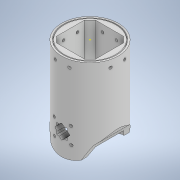
# Autodesk Inventor part: brazo_base_1
Saved by Autodesk Inventor 2021 (Build 250183000, 183)
## iProperties
Created: 2021-03-15
Part Number: brazo_base_1
Material: Genérico
Document SubType Name: Modeling
Designer: Joaquín
Density: 1 g/cm^3
Appearance: Valor por defecto
Author: Joaquín
Autodesk Inventor part; units mm, degrees
ref_plane "YZ Plane" through (0, 0, 0) normal (1, 0, 0) x (0, 1, 0)
ref_plane "XZ Plane" through (0, 0, 0) normal (0, 1, 0) x (-1, 0, 0)
ref_plane "XY Plane" through (0, 0, 0) normal (0, 0, 1) x (1, 0, 0)
sketch "Boceto4" plane through (0, 0, 0) normal (0, 1, 0) x (-1, 0, 0)
  line L0 (-22.5, 0) -> (-22.5, -16)
  line L1 (0, -22.5) -> (-16, -22.5)
  line L2 (-16, -22.5) -> (-22.5, -16)
  line L3 (0, -22.5) -> (16, -22.5)
  line L4 (22.5, 0) -> (22.5, -16)
  line L5 (22.5, -16) -> (16, -22.5)
  line L6 (22.5, 0) -> (22.5, 16)
  line L7 (0, 22.5) -> (16, 22.5)
  line L8 (16, 22.5) -> (22.5, 16)
  line L9 (0, 22.5) -> (-16, 22.5)
  line L10 (-22.5, 0) -> (-22.5, 16)
  line L11 (-22.5, 16) -> (-16, 22.5)
  line L12 (-16, 25) -> (16, 25)
  line L13 (25, 16) -> (25, -16)
  line L14 (16, -25) -> (-16, -25)
  line L15 (-25, -16) -> (-25, 16)
  line L16 (16, -25) -> (25, -16)
  line L17 (25, 16) -> (16, 25)
  line L18 (-25, 16) -> (-16, 25)
  line L19 (-25, -16) -> (-16, -25)
  point P0 (0, 0)
  dimension "d22" = 360
  constraints: 40 end point, 3 parallel, 1 horizontal, 1 perpendicular, 29 other
extrude "Extrusión2" add sketch "Boceto4" along normal blind 100
sketch "Boceto5" plane through (0, 0, 0) normal (0, -1, 0) x (1, 0, 0)
  circle A0 centre (0, 0) radius 32.5
  line L0 (-25, -16) -> (-25, 16) projected
  line L1 (-25, 16) -> (-16, 25) projected
  line L2 (-25, 16) -> (-16, 25)
  line L3 (-16, 25) -> (16, 25)
  line L4 (16, 25) -> (25, 16) projected
  line L5 (16, 25) -> (25, 16)
  line L6 (25, 16) -> (25, -16) projected
  line L7 (25, 16) -> (25, -16)
  line L8 (25, -16) -> (16, -25)
  line L9 (16, -25) -> (-16, -25) projected
  line L10 (16, -25) -> (-16, -25)
  line L11 (-16, -25) -> (-25, -16)
  line L12 (-25, -16) -> (-25, 16)
  constraints: 16 end point, 6 equal length, 1 centre point, 1 coincident, 1 horizontal, 1 perpendicular
sketch "Boceto6" plane through (-16, 0, 25) normal (0, 0, 1) x (1, 0, 0)
  line L0 (13, 19) -> (10, 19)
  line L1 (10, 31) -> (13, 31)
  line L2 (10, 31) -> (10, 28)
  line L3 (22, 19) -> (22, 22)
  line L4 (7.5147, 25) -> (10, 22)
  line L5 (13, 19) -> (16, 16.5147)
  line L6 (19, 19) -> (16, 16.5147)
  line L7 (22, 22) -> (24.4853, 25)
  line L8 (24.4853, 25) -> (22, 28)
  line L9 (19, 31) -> (16, 33.4853)
  line L10 (16, 33.4853) -> (13, 31)
  line L11 (10, 28) -> (7.5147, 25)
  line L12 (10, 31) -> (10, 28)
  line L13 (10, 22) -> (10, 19)
  line L14 (10, 19) -> (13, 19)
  line L15 (19, 19) -> (22, 19)
  line L16 (22, 19) -> (22, 22)
  line L17 (22, 28) -> (22, 31)
  line L18 (19, 31) -> (22, 31)
  point P0 (16, 0)
  constraints: 38 end point, 4 parallel, 4 perpendicular, 3 horizontal
sketch "Boceto7" plane through (-16, 0, 25) normal (0, 0, 1) x (1, 0, 0)
  line L0 (-9, 18) -> (-1.4121, 2.8243)
  line L1 (41, 0) -> (41, 100) projected
  line L2 (32, 0) -> (32, 100) projected
  line L3 (33.4121, 2.8243) -> (41, 18)
  line L4 (-9, 0) -> (-9, 100) projected
  line L5 (-19, 18) -> (-19, 0)
  line L6 (51, 18) -> (51, 0)
  line L7 (-9, 0) -> (-9, 10)
  line L8 (-9, 0) -> (-9, 100) projected
  line L9 (41, 0) -> (41, 10)
  line L10 (41, 10) -> (-9, 10)
  line L11 (-9, 10) -> (16, 10)
  ellipse E0 centre (16, 10) end of major axis (-9, 10) minor radius 10 (-1.4121, 2.8243) -> (33.4121, 2.8243) ccw
  line L12 (0, 0) -> (0, 100) projected
  line L13 (-19, 0) -> (16, 0)
  line L14 (16, 0) -> (51, 0)
  line L15 (32, 0) -> (0, 0) projected
  line L16 (-19, 18) -> (-19, 38)
  line L17 (51, 18) -> (51, 38)
  arc A0 (-19, 38) -> (-9, 18) centre (10.8998, 40.4499) ccw
  arc A1 (41, 18) -> (51, 38) centre (21.1002, 40.4499) ccw
  point P0 (32, 2.3163)
  dimension "d53" = 10
  dimension "d54" = 10
  dimension "d55" = 25
  dimension "d58" = 20
  dimension "d59" = 20
  dimension "d60" = 30
  dimension "d61" = 30
  constraints: 24 end point, 4 point on circle, 4 point on line, 2 centre point, 2 horizontal, 2 vertical, 1 coincident, 1 collinear, 1 midpoint, 5 other
  measures "d53" distance of L7.end L4.start
  measures "d54" distance of L1.start L9.end
  measures "d55" distance of L7.end L11.end
  measures "d58" distance of L5.start L16.end
  measures "d59" distance of L6.start L17.end
  measures "d60" radius of A0
  measures "d61" radius of A1
extrude "Extrusión4" add sketch "Boceto5" against normal blind 100
extrude "Extrusión8" cut sketch "Boceto7" against normal mid plane 200 contours L0 L10 L4 | L4 L13 L5 L16 A0 | L0 E0 L12 L13 L4 L10 | E0 L13 L12 | E0 L2 L14 | E0 L3 L10 L1 L14 L2 | L3 L1 L10 | L1 A1 L17 L6 L14
extrude "Extrusión10" cut sketch "Boceto6" against normal mid plane 200
sketch "Boceto10" plane through (-16, 100, -22.5) normal (0, 0, 1) x (1, 0, 0)
  line L0 (0, 0) -> (8, 0)
  line L1 (0, 0) -> (32, 0) projected
  line L2 (8, 0) -> (8, -8)
  circle A0 centre (8, -8) radius 1.5
  line L3 (32, -97.6837) -> (32, 0) projected
  line L4 (32, 0) -> (24, 0)
  line L5 (24, 0) -> (24, -8)
  circle A1 centre (24, -8) radius 1.5
  point P0 (16, -100)
  dimension "d95" = 8
  dimension "d96" = 8
  dimension "d97" = 3
  dimension "d98" = 8
  dimension "d99" = 8
  dimension "d100" = 3
  constraints: 8 end point, 2 centre point, 2 coincident, 2 perpendicular, 2 point on line
  measures "d95" distance of L0.start L0.end
  measures "d96" distance of L0.end L2.end
  measures "d97" diameter of A0
  measures "d98" distance of L1.end L4.end
  measures "d99" distance of L4.end L5.end
  measures "d100" diameter of A1
extrude "Extrusión12" cut sketch "Boceto10" along normal mid plane 200
sketch "Boceto11" plane through (22.5, 100, -16) normal (-1, 0, 0) x (0, 0, 1)
  circle A0 centre (8, -8) radius 1.5
  circle A1 centre (24, -8) radius 1.5
  point P0 (16, -100)
  point P1 (0, 0)
  point P2 (32, 0)
  constraints: 2 centre point
extrude "Extrusión13" cut sketch "Boceto11" against normal mid plane 200
sketch "Boceto12" plane through (0, 100, 0) normal (0, 1, 0) x (1, 0, 0)
  circle A0 centre (0, 0) radius 29.5
  circle A1 centre (0, 0) radius 30.5
  dimension "d113" = 59
  dimension "d114" = 61
  constraints: 2 centre point, 2 coincident
  measures "d113" diameter of A0
  measures "d114" diameter of A1
extrude "Extrusión14" cut sketch "Boceto12" against normal blind 2.5
sketch "Boceto13" plane through (16, 100, 22.5) normal (0, 0, -1) x (-1, 0, 0)
  line L0 (19, -69) -> (16, -66.5147) projected
  line L1 (19, -81) -> (16, -83.4853) projected
  line L2 (16, -66.5147) -> (16, -83.4853)
  line L3 (22, -72) -> (24.4853, -75) projected
  line L4 (7.5147, -75) -> (10, -72) projected
  line L5 (24.4853, -75) -> (7.5147, -75)
  line L6 (10, -72) -> (10, -69) projected
  line L7 (22, -81) -> (19, -81) projected
  line L8 (10, -69) -> (22, -81)
  circle A0 centre (25.3117, -84.6846) radius 1.5
  circle A1 centre (25.6846, -65.6883) radius 1.5
  circle A2 centre (6.6883, -65.3154) radius 1.5
  circle A3 centre (6.3154, -84.3117) radius 1.5
  point P0 (16, -100)
  point P1 (16, -75)
  dimension "d121" = 360
  constraints: 6 end point, 4 centre point, 1 horizontal, 1 midpoint, 1 vertical, 9 other
extrude "Extrusión15" cut sketch "Boceto13" against normal mid plane 200 contours A0 | A1 | A2 | A3
sketch "Boceto14" plane through (0, 100, 0) normal (0, 1, 0) x (1, 0, 0)
  point P0 (0, 0)
